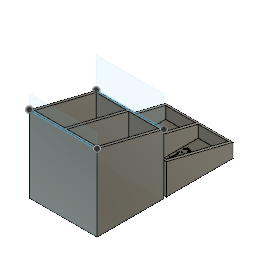
DeckBox (Autodesk Fusion 360 design; units mm, degrees)
Autodesk Fusion 360 part; units mm, degrees
(part 1 of 5)
sketch "Sketch1" plane through (0, 0, 0) normal (0, 0, 1) x (1, 0, 0)
  line L0 (0, 0) -> (35, 0)
  line L1 (35, 0) -> (35, 72)
  line L2 (35, 72) -> (0, 72)
  line L3 (0, 72) -> (0, 0)
  line L4 (38, 0) -> (73, 0)
  line L5 (73, 0) -> (73, 72)
  line L6 (73, 72) -> (38, 72)
  line L7 (38, 72) -> (38, 0)
  line L8 (0, 72) -> (-3, 72)
  line L9 (-3, 72) -> (-3, 75)
  line L10 (-3, 75) -> (0, 75)
  line L11 (0, 75) -> (0, 72)
  line L12 (73, 0) -> (76, 0)
  line L13 (76, 0) -> (76, -3)
  line L14 (76, -3) -> (73, -3)
  line L15 (73, -3) -> (73, 0)
  line L16 (-3, 75) -> (76, 75)
  line L17 (76, 75) -> (76, -3)
  line L18 (76, -3) -> (-3, -3)
  line L19 (-3, -3) -> (-3, 75)
  dimension "d5" = 35
  dimension "d6" = 72
  dimension "d7" = 35
  dimension "d8" = 72
  dimension "d9" = 3
  dimension "d10" = 3
  dimension "d11" = 3
  dimension "d12" = 3
  constraint horizontal L0
  constraint vertical L1
  constraint horizontal L2
  constraint vertical L3
  constraint coincident L0.start L3.end
  constraint horizontal L4
  constraint vertical L5
  constraint horizontal L6
  constraint vertical L7
  constraint horizontal L8
  constraint vertical L9
  constraint horizontal L10
  constraint vertical L11
  constraint horizontal L12
  constraint vertical L13
  constraint horizontal L14
  constraint vertical L15
  constraint horizontal L16
  constraint vertical L17
  constraint horizontal L18
  constraint vertical L19
  measures "d5" distance of L0.start L0.end
  measures "d6" distance of L0.start L2.end
  measures "d7" distance of L4.start L4.end
  measures "d8" distance of L4.start L6.end
  measures "d9" distance of L2.end L8.end
  measures "d10" distance of L2.end L10.end
  measures "d11" distance of L4.end L12.end
  measures "d12" distance of L4.end L14.end
extrude "Extrude1" add sketch "Sketch1" along normal blind 106 makes body 1
sketch "Sketch2" plane through (0, -3, 0) normal (0, -1, 0) x (1, 0, 0)
  line L0 (-3, 0) -> (76, 0)
  line L1 (76, 0) -> (76, 106)
  line L2 (76, 106) -> (-3, 106)
  line L3 (-3, 106) -> (-3, 0)
  line L4 (-3, 106) -> (76, 106)
  line L5 (76, 106) -> (76, 103)
  line L6 (76, 103) -> (-3, 103)
  line L7 (-3, 103) -> (-3, 106)
  line L8 (-3, 0) -> (76, 0)
  line L9 (76, 0) -> (76, 3)
  line L10 (76, 3) -> (-3, 3)
  line L11 (-3, 3) -> (-3, 0)
  dimension "d15" = 3
  dimension "d16" = 3
  constraint horizontal L4
  constraint vertical L5
  constraint horizontal L6
  constraint vertical L7
  constraint coincident L2.end L3.start
  constraint horizontal L8
  constraint vertical L9
  constraint horizontal L10
  constraint vertical L11
  constraint coincident L0.start L3.end
  measures "d15" distance of L2.end L6.end
  measures "d16" distance of L0.start L10.end
extrude "Extrude2" add sketch "Sketch2" against normal blind 78 contours L1 L2 L3 L4 L5 L6 L7 bodies 1
sketch "Sketch3" plane through (0, -3, 0) normal (0, -1, 0) x (1, 0, 0)
  line L0 (-3, 106) -> (-3, 0)
  line L1 (-3, 0) -> (76, 0)
  line L2 (76, 0) -> (76, 106)
  line L3 (76, 106) -> (-3, 106)
  line L4 (-3, 89.5775) -> (76, 89.5775)
  constraint coincident L0 L4.start
  constraint coincident L2 L4.end
  constraint perpendicular L2 L4
sketch "Sketch4" plane through (0, 75, 0) normal (0, 1, 0) x (-1, 0, 0)
  line L0 (-76, 106) -> (-76, 0)
  line L1 (-76, 0) -> (3, 0)
  line L2 (3, 0) -> (3, 106)
  line L3 (3, 106) -> (-76, 106)
  line L4 (-76, 70.2322) -> (3, 70.2322)
  constraint coincident L0 L4.start
  constraint coincident L2 L4.end
  constraint perpendicular L2 L4
ref_plane "WorkPlane1" through (-3, -3, 89.5775) normal (0, -0.240723, -0.970594) x (1, 0, 0)
split "Split1" by plane through (-3, -3, 89.5775) normal (0, -0.240723, -0.970594) bodies 1 makes body 2 at (49.6667, -3, 59.7183)
move_body "Move1" bodies 1 to x (1, 0, 0) y (0, -1, 0) z (0, 0, -1) at (0, 153.0762, 106.2506)
sketch "Sketch5" plane through (76, 0, 0) normal (1, 0, 0) x (0, 1, 0)
  line L0 (75, 70.2322) -> (-3, 89.5775)
  line L1 (-3, 89.5775) -> (-3, 0)
  line L2 (-3, 0) -> (75, 0)
  line L3 (75, 0) -> (75, 70.2322)
  line L4 (-3, 0) -> (75, 0)
  line L5 (75, 0) -> (75, 3)
  line L6 (75, 3) -> (-3, 3)
  line L7 (-3, 3) -> (-3, 0)
  dimension "d19" = 3
  constraint horizontal L4
  constraint vertical L5
  constraint horizontal L6
  constraint vertical L7
  constraint coincident L3 L5.end
  constraint coincident L1.end L2.start
  measures "d19" distance of L1.end L6.end
extrude "Extrude3" add sketch "Sketch5" against normal blind 79 contours L1 L2 L3 L4 L5 L6 L7 bodies 2
sketch "Sketch6" plane through (0, 0, 3.2506) normal (0, 0, 1) x (-1, 0, 0)
  line L0 (-73, -153.0762) -> (-38, -153.0762)
  line L1 (-38, -153.0762) -> (-38, -81.0762)
  line L2 (-38, -81.0762) -> (-73, -81.0762)
  line L3 (-73, -81.0762) -> (-73, -153.0762)
  spline S0 degree 3 poles (-57.9269, -101.8544) (-58.3701, -102.5297) (-58.3595, -103.2367) (-57.8847, -103.6377) knots 0 0 0 0 1 1 1 1
  line L4 (-57.8847, -103.6377) -> (-57.5892, -103.8804)
  line L5 (-57.5892, -103.8804) -> (-58.3384, -104.0703)
  spline S1 degree 3 poles (-58.3384, -104.0703) (-58.75, -104.1758) (-59.2881, -104.3763) (-59.5308, -104.503) knots 0 0 0 0 1 1 1 1
  line L6 (-59.5308, -104.503) -> (-59.9846, -104.7457)
  line L7 (-59.9846, -104.7457) -> (-60.5333, -104.2286)
  spline S2 degree 3 poles (-60.5333, -104.2286) (-61.1031, -103.701) (-61.3036, -103.6166) (-61.388, -103.8382) knots 0 0 0 0 1 1 1 1
  spline S3 degree 3 poles (-61.388, -103.8382) (-61.4196, -103.9437) (-61.4935, -103.9437) (-61.6834, -103.8276) knots 0 0 0 0 1 1 1 1
  spline S4 degree 3 poles (-61.6834, -103.8276) (-62.1688, -103.5322) (-63.5722, -103.3) (-64.5219, -103.3422) knots 0 0 0 0 1 1 1 1
  spline S5 degree 3 poles (-64.5219, -103.3422) (-65.7565, -103.4055) (-65.957, -103.4478) (-66.4318, -103.7538) knots 0 0 0 0 1 1 1 1
  spline S6 degree 3 poles (-66.4318, -103.7538) (-67.0228, -104.1442) (-67.2233, -104.619) (-67.2866, -105.7164) knots 0 0 0 0 1 1 1 1
  spline S7 degree 3 poles (-67.2866, -105.7164) (-67.3077, -106.1174) (-67.4026, -106.2968) (-67.8669, -106.8666) knots 0 0 0 0 1 1 1 1
  spline S8 degree 3 poles (-67.8669, -106.8666) (-68.1729, -107.2465) (-68.4262, -107.6158) (-68.4262, -107.6791) knots 0 0 0 0 1 1 1 1
  spline S9 degree 3 poles (-68.4262, -107.6791) (-68.4262, -107.753) (-68.7216, -108.0379) (-69.0804, -108.3122) knots 0 0 0 0 1 1 1 1
  spline S10 degree 3 poles (-69.0804, -108.3122) (-70.5049, -109.378) (-71.4546, -110.6653) (-71.6446, -111.7733) knots 0 0 0 0 1 1 1 1
  spline S11 degree 3 poles (-71.6446, -111.7733) (-71.7079, -112.1532) (-71.6973, -112.1848) (-71.539, -112.0477) knots 0 0 0 0 1 1 1 1
  spline S12 degree 3 poles (-71.539, -112.0477) (-71.4335, -111.9632) (-71.3913, -111.8155) (-71.423, -111.6889) knots 0 0 0 0 1 1 1 1
  spline S13 degree 3 poles (-71.423, -111.6889) (-71.5601, -111.1613) (-70.3572, -109.589) (-69.1121, -108.671) knots 0 0 0 0 1 1 1 1
  spline S14 degree 3 poles (-69.1121, -108.671) (-68.5317, -108.2489) (-67.3815, -107.563) (-67.3393, -107.6264) knots 0 0 0 0 1 1 1 1
  spline S15 degree 3 poles (-67.3393, -107.6264) (-67.3182, -107.6475) (-67.2444, -107.7846) (-67.1705, -107.9324) knots 0 0 0 0 1 1 1 1
  spline S16 degree 3 poles (-67.1705, -107.9324) (-67.1072, -108.0801) (-66.8856, -108.4811) (-66.7062, -108.8293) knots 0 0 0 0 1 1 1 1
  line L8 (-66.7062, -108.8293) -> (-66.3685, -109.4624)
  line L9 (-66.3685, -109.4624) -> (-67.2655, -110.1588)
  spline S17 degree 3 poles (-67.2655, -110.1588) (-67.7614, -110.5387) (-68.5634, -111.2774) (-69.0382, -111.7839) knots 0 0 0 0 1 1 1 1
  spline S18 degree 3 poles (-69.0382, -111.7839) (-69.513, -112.2904) (-69.9035, -112.6386) (-69.9035, -112.5542) knots 0 0 0 0 1 1 1 1
  spline S19 degree 3 poles (-69.9035, -112.5542) (-69.9035, -112.1954) (-69.4392, -110.9502) (-69.1226, -110.486) knots 0 0 0 0 1 1 1 1
  spline S20 degree 3 poles (-69.1226, -110.486) (-68.8272, -110.0428) (-68.7427, -109.99) (-68.1835, -109.8739) knots 0 0 0 0 1 1 1 1
  spline S21 degree 3 poles (-68.1835, -109.8739) (-67.4871, -109.7368) (-67.2127, -109.5574) (-67.8458, -109.6523) knots 0 0 0 0 1 1 1 1
  spline S22 degree 3 poles (-67.8458, -109.6523) (-69.1543, -109.8528) (-70.3467, -110.4015) (-71.0536, -111.1402) knots 0 0 0 0 1 1 1 1
  spline S23 degree 3 poles (-71.0536, -111.1402) (-71.5601, -111.6678) (-71.4124, -111.71) (-70.8531, -111.2035) knots 0 0 0 0 1 1 1 1
  spline S24 degree 3 poles (-70.8531, -111.2035) (-70.4733, -110.8553) (-69.3864, -110.2116) (-69.3126, -110.2855) knots 0 0 0 0 1 1 1 1
  spline S25 degree 3 poles (-69.3126, -110.2855) (-69.2914, -110.296) (-69.4181, -110.5915) (-69.5869, -110.9397) knots 0 0 0 0 1 1 1 1
  spline S26 degree 3 poles (-69.5869, -110.9397) (-69.7557, -111.2879) (-69.9351, -111.8577) (-69.9984, -112.1954) knots 0 0 0 0 1 1 1 1
  spline S27 degree 3 poles (-69.9984, -112.1954) (-70.0934, -112.6913) (-70.2728, -113.0712) (-70.9059, -114.0314) knots 0 0 0 0 1 1 1 1
  spline S28 degree 3 poles (-70.9059, -114.0314) (-71.3385, -114.6962) (-71.6973, -115.3399) (-71.6973, -115.4665) knots 0 0 0 0 1 1 1 1
  spline S29 degree 3 poles (-71.6973, -115.4665) (-71.6973, -115.6353) (-71.634, -115.5826) (-71.4441, -115.2449) knots 0 0 0 0 1 1 1 1
  spline S30 degree 3 poles (-71.4441, -115.2449) (-70.4944, -113.5777) (-68.3734, -111.1402) (-66.9172, -110.0533) knots 0 0 0 0 1 1 1 1
  spline S31 degree 3 poles (-66.9172, -110.0533) (-66.4107, -109.6735) (-66.2841, -109.6207) (-66.1575, -109.7262) knots 0 0 0 0 1 1 1 1
  spline S32 degree 3 poles (-66.1575, -109.7262) (-66.0098, -109.8423) (-66.0098, -109.8845) (-66.1786, -110.0639) knots 0 0 0 0 1 1 1 1
  spline S33 degree 3 poles (-66.1786, -110.0639) (-66.3369, -110.2433) (-66.3474, -110.2855) (-66.2103, -110.3699) knots 0 0 0 0 1 1 1 1
  spline S34 degree 3 poles (-66.2103, -110.3699) (-65.746, -110.6442) (-65.7565, -110.602) (-66.0836, -111.6572) knots 0 0 0 0 1 1 1 1
  spline S35 degree 3 poles (-66.0836, -111.6572) (-66.7379, -113.6938) (-67.7086, -115.878) (-68.194, -116.3951) knots 0 0 0 0 1 1 1 1
  spline S36 degree 3 poles (-68.194, -116.3951) (-68.3418, -116.5639) (-68.4367, -116.6906) (-68.3945, -116.6906) knots 0 0 0 0 1 1 1 1
  spline S37 degree 3 poles (-68.3945, -116.6906) (-68.194, -116.6906) (-67.3499, -116.2157) (-66.9911, -115.9097) knots 0 0 0 0 1 1 1 1
  line L10 (-66.9911, -115.9097) -> (-66.5796, -115.5615)
  line L11 (-66.5796, -115.5615) -> (-66.5901, -117.2076)
  spline S38 degree 3 poles (-66.5901, -117.2076) (-66.6112, -120.0039) (-66.8961, -120.9958) (-67.8458, -121.6289) knots 0 0 0 0 1 1 1 1
  spline S39 degree 3 poles (-67.8458, -121.6289) (-68.2046, -121.861) (-68.2785, -121.956) (-68.1518, -122.0088) knots 0 0 0 0 1 1 1 1
  spline S40 degree 3 poles (-68.1518, -122.0088) (-67.8458, -122.1248) (-67.1072, -122.0615) (-66.5585, -121.8716) knots 0 0 0 0 1 1 1 1
  line L12 (-66.5585, -121.8716) -> (-66.0098, -121.6922)
  line L13 (-66.0098, -121.6922) -> (-66.2841, -122.2198)
  spline S41 degree 3 poles (-66.2841, -122.2198) (-66.4318, -122.5153) (-66.6112, -122.7896) (-66.6745, -122.8318) knots 0 0 0 0 1 1 1 1
  spline S42 degree 3 poles (-66.6745, -122.8318) (-66.9911, -123.0429) (-66.1153, -122.8846) (-65.7354, -122.663) knots 0 0 0 0 1 1 1 1
  line L14 (-65.7354, -122.663) -> (-65.3028, -122.3992)
  line L15 (-65.3028, -122.3992) -> (-65.1762, -123.2117)
  spline S43 degree 3 poles (-65.1762, -123.2117) (-65.1128, -123.6549) (-64.8807, -124.478) (-64.6697, -125.0267) knots 0 0 0 0 1 1 1 1
  spline S44 degree 3 poles (-64.6697, -125.0267) (-64.2054, -126.2612) (-64.0154, -126.926) (-63.931, -127.6119) knots 0 0 0 0 1 1 1 1
  spline S45 degree 3 poles (-63.931, -127.6119) (-63.8783, -128.1078) (-63.8994, -128.1712) (-64.3214, -128.7515) knots 0 0 0 0 1 1 1 1
  spline S46 degree 3 poles (-64.3214, -128.7515) (-64.5641, -129.0786) (-64.8068, -129.353) (-64.849, -129.353) knots 0 0 0 0 1 1 1 1
  spline S47 degree 3 poles (-64.849, -129.353) (-65.0284, -129.353) (-65.039, -129.1631) (-64.8913, -128.6671) knots 0 0 0 0 1 1 1 1
  spline S48 degree 3 poles (-64.8913, -128.6671) (-64.7119, -128.0762) (-64.6697, -127.116) (-64.849, -127.5486) knots 0 0 0 0 1 1 1 1
  spline S49 degree 3 poles (-64.849, -127.5486) (-64.9018, -127.6858) (-65.2817, -128.129) (-65.6827, -128.5299) knots 0 0 0 0 1 1 1 1
  spline S50 degree 3 poles (-65.6827, -128.5299) (-66.2525, -129.0997) (-66.4635, -129.2475) (-66.6218, -129.1947) knots 0 0 0 0 1 1 1 1
  spline S51 degree 3 poles (-66.6218, -129.1947) (-66.9067, -129.1103) (-67.6664, -129.3108) (-68.0358, -129.5746) knots 0 0 0 0 1 1 1 1
  spline S52 degree 3 poles (-68.0358, -129.5746) (-68.2046, -129.7012) (-68.3629, -129.7751) (-68.384, -129.7434) knots 0 0 0 0 1 1 1 1
  spline S53 degree 3 poles (-68.384, -129.7434) (-68.4473, -129.6907) (-68.1202, -128.9415) (-67.4026, -127.4747) knots 0 0 0 0 1 1 1 1
  spline S54 degree 3 poles (-67.4026, -127.4747) (-67.0755, -126.8205) (-66.8434, -126.2612) (-66.875, -126.2296) knots 0 0 0 0 1 1 1 1
  spline S55 degree 3 poles (-66.875, -126.2296) (-66.9067, -126.1979) (-67.1283, -126.5884) (-67.3815, -127.0949) knots 0 0 0 0 1 1 1 1
  spline S56 degree 3 poles (-67.3815, -127.0949) (-67.9513, -128.2872) (-68.4684, -128.7937) (-69.5025, -129.2264) knots 0 0 0 0 1 1 1 1
  spline S57 degree 3 poles (-69.5025, -129.2264) (-70.5577, -129.6695) (-70.6632, -129.6484) (-70.0406, -129.1525) knots 0 0 0 0 1 1 1 1
  spline S58 degree 3 poles (-70.0406, -129.1525) (-69.7663, -128.9309) (-69.4075, -128.6143) (-69.2598, -128.4455) knots 0 0 0 0 1 1 1 1
  spline S59 degree 3 poles (-69.2598, -128.4455) (-68.8377, -127.9707) (-68.1624, -126.8311) (-67.9091, -126.1452) knots 0 0 0 0 1 1 1 1
  spline S60 degree 3 poles (-67.9091, -126.1452) (-67.7825, -125.797) (-67.6453, -125.4698) (-67.6031, -125.4065) knots 0 0 0 0 1 1 1 1
  spline S61 degree 3 poles (-67.6031, -125.4065) (-67.5715, -125.3432) (-67.5293, -125.2377) (-67.5187, -125.1849) knots 0 0 0 0 1 1 1 1
  spline S62 degree 3 poles (-67.5187, -125.1849) (-67.5082, -125.1216) (-67.3815, -124.7101) (-67.2233, -124.2564) knots 0 0 0 0 1 1 1 1
  spline S63 degree 3 poles (-67.2233, -124.2564) (-67.0755, -123.8026) (-66.9067, -123.2328) (-66.8434, -122.9796) knots 0 0 0 0 1 1 1 1
  spline S64 degree 3 poles (-66.8434, -122.9796) (-66.7906, -122.7369) (-66.7168, -122.452) (-66.6745, -122.357) knots 0 0 0 0 1 1 1 1
  spline S65 degree 3 poles (-66.6745, -122.357) (-66.6429, -122.262) (-66.6534, -122.1776) (-66.7062, -122.1776) knots 0 0 0 0 1 1 1 1
  spline S66 degree 3 poles (-66.7062, -122.1776) (-66.759, -122.1776) (-66.8856, -122.5469) (-66.9911, -122.9901) knots 0 0 0 0 1 1 1 1
  spline S67 degree 3 poles (-66.9911, -122.9901) (-67.0966, -123.4439) (-67.2233, -123.8554) (-67.2655, -123.9187) knots 0 0 0 0 1 1 1 1
  spline S68 degree 3 poles (-67.2655, -123.9187) (-67.2971, -123.9715) (-67.4871, -124.4991) (-67.6875, -125.0794) knots 0 0 0 0 1 1 1 1
  spline S69 degree 3 poles (-67.6875, -125.0794) (-68.0674, -126.2401) (-68.4895, -127.1687) (-68.8799, -127.6858) knots 0 0 0 0 1 1 1 1
  spline S70 degree 3 poles (-68.8799, -127.6858) (-69.0171, -127.8757) (-69.1648, -128.1184) (-69.1965, -128.2134) knots 0 0 0 0 1 1 1 1
  spline S71 degree 3 poles (-69.1965, -128.2134) (-69.2809, -128.4455) (-70.6738, -129.4691) (-71.2436, -129.7223) knots 0 0 0 0 1 1 1 1
  spline S72 degree 3 poles (-71.2436, -129.7223) (-71.4968, -129.8278) (-71.6973, -129.9545) (-71.6973, -130.0072) knots 0 0 0 0 1 1 1 1
  spline S73 degree 3 poles (-71.6973, -130.0072) (-71.6973, -130.1338) (-71.5179, -130.1127) (-71.1908, -129.9439) knots 0 0 0 0 1 1 1 1
  spline S74 degree 3 poles (-71.1908, -129.9439) (-71.0325, -129.87) (-70.6738, -129.7645) (-70.3889, -129.7223) knots 0 0 0 0 1 1 1 1
  spline S75 degree 3 poles (-70.3889, -129.7223) (-69.7346, -129.6273) (-68.901, -129.2686) (-68.4367, -128.8676) knots 0 0 0 0 1 1 1 1
  line L16 (-68.4367, -128.8676) -> (-68.0674, -128.5616)
  line L17 (-68.0674, -128.5616) -> (-68.3734, -129.1314)
  line L18 (-68.3734, -129.1314) -> (-68.6794, -129.6907)
  line L19 (-68.6794, -129.6907) -> (-69.1332, -129.6273)
  spline S76 degree 3 poles (-69.1332, -129.6273) (-69.608, -129.564) (-69.6713, -129.6273) (-69.4919, -129.9756) knots 0 0 0 0 1 1 1 1
  spline S77 degree 3 poles (-69.4919, -129.9756) (-69.4075, -130.1338) (-69.4708, -130.2077) (-69.8929, -130.4398) knots 0 0 0 0 1 1 1 1
  spline S78 degree 3 poles (-69.8929, -130.4398) (-70.2939, -130.6509) (-71.6973, -131.9171) (-71.6973, -132.0649) knots 0 0 0 0 1 1 1 1
  spline S79 degree 3 poles (-71.6973, -132.0649) (-71.6973, -132.2231) (-71.3913, -131.991) (-70.832, -131.4106) knots 0 0 0 0 1 1 1 1
  spline S80 degree 3 poles (-70.832, -131.4106) (-70.3467, -130.9041) (-70.0195, -130.672) (-69.6186, -130.5243) knots 0 0 0 0 1 1 1 1
  spline S81 degree 3 poles (-69.6186, -130.5243) (-69.1543, -130.3554) (-69.0488, -130.3449) (-68.9432, -130.4715) knots 0 0 0 0 1 1 1 1
  spline S82 degree 3 poles (-68.9432, -130.4715) (-68.8799, -130.5559) (-68.7216, -130.6192) (-68.595, -130.6192) knots 0 0 0 0 1 1 1 1
  spline S83 degree 3 poles (-68.595, -130.6192) (-68.4051, -130.6192) (-68.4156, -130.5981) (-68.69, -130.4187) knots 0 0 0 0 1 1 1 1
  spline S84 degree 3 poles (-68.69, -130.4187) (-68.8588, -130.3132) (-69.1015, -130.1233) (-69.207, -129.9967) knots 0 0 0 0 1 1 1 1
  line L20 (-69.207, -129.9967) -> (-69.4075, -129.7751)
  line L21 (-69.4075, -129.7751) -> (-68.8905, -129.8384)
  spline S85 degree 3 poles (-68.8905, -129.8384) (-68.6056, -129.8806) (-68.3523, -129.9228) (-68.3312, -129.9545) knots 0 0 0 0 1 1 1 1
  spline S86 degree 3 poles (-68.3312, -129.9545) (-68.2996, -129.9756) (-68.1835, -129.9017) (-68.0674, -129.7856) knots 0 0 0 0 1 1 1 1
  spline S87 degree 3 poles (-68.0674, -129.7856) (-67.5609, -129.3319) (-66.5585, -129.258) (-65.862, -129.6168) knots 0 0 0 0 1 1 1 1
  line L22 (-65.862, -129.6168) -> (-65.5771, -129.7645)
  line L23 (-65.5771, -129.7645) -> (-65.6404, -129.3424)
  line L24 (-65.6404, -129.3424) -> (-65.7143, -128.9204)
  line L25 (-65.7143, -128.9204) -> (-65.3344, -129.1631)
  spline S88 degree 3 poles (-65.3344, -129.1631) (-65.1234, -129.3002) (-64.9546, -129.4269) (-64.9546, -129.4585) knots 0 0 0 0 1 1 1 1
  spline S89 degree 3 poles (-64.9546, -129.4585) (-64.944, -129.5746) (-65.8726, -130.176) (-66.2419, -130.3027) knots 0 0 0 0 1 1 1 1
  spline S90 degree 3 poles (-66.2419, -130.3027) (-66.7906, -130.4715) (-66.6323, -130.6614) (-65.9887, -130.5876) knots 0 0 0 0 1 1 1 1
  spline S91 degree 3 poles (-65.9887, -130.5876) (-65.4822, -130.5243) (-64.733, -130.2077) (-64.3848, -129.9017) knots 0 0 0 0 1 1 1 1
  spline S92 degree 3 poles (-64.3848, -129.9017) (-64.2687, -129.7962) (-64.3425, -130.0494) (-64.6063, -130.6298) knots 0 0 0 0 1 1 1 1
  spline S93 degree 3 poles (-64.6063, -130.6298) (-64.8385, -131.1152) (-65.0495, -131.59) (-65.0812, -131.685) knots 0 0 0 0 1 1 1 1
  spline S94 degree 3 poles (-65.0812, -131.685) (-65.1128, -131.78) (-65.3344, -131.9488) (-65.5666, -132.0543) knots 0 0 0 0 1 1 1 1
  spline S95 degree 3 poles (-65.5666, -132.0543) (-65.7987, -132.1704) (-65.9992, -132.2865) (-65.9992, -132.3287) knots 0 0 0 0 1 1 1 1
  spline S96 degree 3 poles (-65.9992, -132.3287) (-65.9992, -132.4025) (-65.862, -132.3603) (-65.2078, -132.086) knots 0 0 0 0 1 1 1 1
  spline S97 degree 3 poles (-65.2078, -132.086) (-65.0284, -132.0121) (-64.8385, -131.9699) (-64.7857, -131.9804) knots 0 0 0 0 1 1 1 1
  spline S98 degree 3 poles (-64.7857, -131.9804) (-64.7224, -132.0015) (-64.7119, -131.9699) (-64.7541, -131.9277) knots 0 0 0 0 1 1 1 1
  spline S99 degree 3 poles (-64.7541, -131.9277) (-64.7963, -131.8855) (-64.5958, -131.6006) (-64.3109, -131.2946) knots 0 0 0 0 1 1 1 1
  spline S100 degree 3 poles (-64.3109, -131.2946) (-63.9521, -130.8936) (-63.7516, -130.5559) (-63.6356, -130.1444) knots 0 0 0 0 1 1 1 1
  spline S101 degree 3 poles (-63.6356, -130.1444) (-63.5406, -129.8278) (-63.4351, -129.4902) (-63.3929, -129.3952) knots 0 0 0 0 1 1 1 1
  spline S102 degree 3 poles (-63.3929, -129.3952) (-63.3507, -129.2791) (-63.3718, -129.2369) (-63.4351, -129.2791) knots 0 0 0 0 1 1 1 1
  spline S103 degree 3 poles (-63.4351, -129.2791) (-63.4984, -129.3213) (-63.625, -129.6379) (-63.7305, -130.0072) knots 0 0 0 0 1 1 1 1
  spline S104 degree 3 poles (-63.7305, -130.0072) (-63.8677, -130.5137) (-64.026, -130.7775) (-64.427, -131.189) knots 0 0 0 0 1 1 1 1
  line L26 (-64.427, -131.189) -> (-64.944, -131.7272)
  line L27 (-64.944, -131.7272) -> (-64.6275, -131.073)
  spline S105 degree 3 poles (-64.6275, -131.073) (-64.4586, -130.7142) (-64.2476, -130.2394) (-64.1526, -130.0178) knots 0 0 0 0 1 1 1 1
  spline S106 degree 3 poles (-64.1526, -130.0178) (-63.9521, -129.5324) (-63.4773, -129.0153) (-63.319, -129.1103) knots 0 0 0 0 1 1 1 1
  spline S107 degree 3 poles (-63.319, -129.1103) (-63.2557, -129.1419) (-63.2346, -129.1419) (-63.2768, -129.0892) knots 0 0 0 0 1 1 1 1
  spline S108 degree 3 poles (-63.2768, -129.0892) (-63.319, -129.047) (-63.2557, -128.8254) (-63.1396, -128.6038) knots 0 0 0 0 1 1 1 1
  spline S109 degree 3 poles (-63.1396, -128.6038) (-63.0235, -128.3716) (-62.9813, -128.1923) (-63.0446, -128.1923) knots 0 0 0 0 1 1 1 1
  spline S110 degree 3 poles (-63.0446, -128.1923) (-63.0974, -128.1923) (-63.1502, -128.2661) (-63.1502, -128.3611) knots 0 0 0 0 1 1 1 1
  spline S111 degree 3 poles (-63.1502, -128.3611) (-63.1502, -128.4561) (-63.4456, -128.8254) (-63.8149, -129.1842) knots 0 0 0 0 1 1 1 1
  spline S112 degree 3 poles (-63.8149, -129.1842) (-64.4903, -129.8595) (-65.345, -130.366) (-65.9992, -130.461) knots 0 0 0 0 1 1 1 1
  line L28 (-65.9992, -130.461) -> (-66.3685, -130.5137)
  line L29 (-66.3685, -130.5137) -> (-66.052, -130.3976)
  spline S113 degree 3 poles (-66.052, -130.3976) (-64.9546, -129.9756) (-63.8888, -128.7199) (-63.3084, -127.1898) knots 0 0 0 0 1 1 1 1
  spline S114 degree 3 poles (-63.3084, -127.1898) (-62.8336, -125.9025) (-62.5382, -123.5705) (-62.8442, -123.3911) knots 0 0 0 0 1 1 1 1
  spline S115 degree 3 poles (-62.8442, -123.3911) (-62.918, -123.3383) (-62.9286, -123.4333) (-62.8864, -123.676) knots 0 0 0 0 1 1 1 1
  spline S116 degree 3 poles (-62.8864, -123.676) (-62.7808, -124.2353) (-63.0235, -125.8181) (-63.3929, -126.9155) knots 0 0 0 0 1 1 1 1
  line L30 (-63.3929, -126.9155) -> (-63.72, -127.9285)
  line L31 (-63.72, -127.9285) -> (-63.7938, -127.4009)
  spline S117 degree 3 poles (-63.7938, -127.4009) (-63.8255, -127.1054) (-63.9943, -126.5145) (-64.1526, -126.0819) knots 0 0 0 0 1 1 1 1
  spline S118 degree 3 poles (-64.1526, -126.0819) (-64.5852, -124.8789) (-64.9229, -123.7288) (-65.0601, -122.9796) knots 0 0 0 0 1 1 1 1
  spline S119 degree 3 poles (-65.0601, -122.9796) (-65.1656, -122.3253) (-65.1656, -122.2937) (-64.8807, -121.8716) knots 0 0 0 0 1 1 1 1
  spline S120 degree 3 poles (-64.8807, -121.8716) (-64.7224, -121.6289) (-64.6275, -121.4073) (-64.6591, -121.3651) knots 0 0 0 0 1 1 1 1
  spline S121 degree 3 poles (-64.6591, -121.3651) (-64.7013, -121.3334) (-64.7646, -121.3968) (-64.8068, -121.5023) knots 0 0 0 0 1 1 1 1
  spline S122 degree 3 poles (-64.8068, -121.5023) (-64.9335, -121.8294) (-65.3872, -122.2831) (-65.8726, -122.568) knots 0 0 0 0 1 1 1 1
  spline S123 degree 3 poles (-65.8726, -122.568) (-66.1258, -122.7158) (-66.3369, -122.8213) (-66.358, -122.8002) knots 0 0 0 0 1 1 1 1
  spline S124 degree 3 poles (-66.358, -122.8002) (-66.3791, -122.7791) (-66.2208, -122.3886) (-65.9992, -121.9349) knots 0 0 0 0 1 1 1 1
  spline S125 degree 3 poles (-65.9992, -121.9349) (-65.7882, -121.4917) (-65.6193, -121.1224) (-65.6404, -121.1224) knots 0 0 0 0 1 1 1 1
  spline S126 degree 3 poles (-65.6404, -121.1224) (-65.6616, -121.1224) (-65.7987, -121.2385) (-65.957, -121.3862) knots 0 0 0 0 1 1 1 1
  spline S127 degree 3 poles (-65.957, -121.3862) (-66.2525, -121.6606) (-66.7062, -121.8188) (-67.4343, -121.8927) knots 0 0 0 0 1 1 1 1
  line L32 (-67.4343, -121.8927) -> (-67.8669, -121.9455)
  line L33 (-67.8669, -121.9455) -> (-67.4343, -121.5023)
  spline S128 degree 3 poles (-67.4343, -121.5023) (-66.8961, -120.9747) (-66.5163, -120.2993) (-66.2314, -119.413) knots 0 0 0 0 1 1 1 1
  spline S129 degree 3 poles (-66.2314, -119.413) (-65.8937, -118.3683) (-65.7882, -117.7985) (-65.7987, -117.197) knots 0 0 0 0 1 1 1 1
  spline S130 degree 3 poles (-65.7987, -117.197) (-65.8093, -116.6906) (-65.8198, -116.7222) (-65.957, -117.5875) knots 0 0 0 0 1 1 1 1
  spline S131 degree 3 poles (-65.957, -117.5875) (-66.0309, -118.1045) (-66.2103, -118.8643) (-66.358, -119.2758) knots 0 0 0 0 1 1 1 1
  spline S132 degree 3 poles (-66.358, -119.2758) (-66.5057, -119.6768) (-66.6007, -119.8456) (-66.5585, -119.6451) knots 0 0 0 0 1 1 1 1
  spline S133 degree 3 poles (-66.5585, -119.6451) (-66.4318, -118.9381) (-66.4213, -118.7376) (-66.4318, -117.6402) knots 0 0 0 0 1 1 1 1
  spline S134 degree 3 poles (-66.4318, -117.6402) (-66.4635, -115.7092) (-66.4318, -115.3927) (-66.2314, -115.1077) knots 0 0 0 0 1 1 1 1
  spline S135 degree 3 poles (-66.2314, -115.1077) (-65.9359, -114.7173) (-65.7671, -114.3691) (-65.862, -114.3691) knots 0 0 0 0 1 1 1 1
  spline S136 degree 3 poles (-65.862, -114.3691) (-65.9148, -114.3691) (-66.0414, -114.5274) (-66.1469, -114.7068) knots 0 0 0 0 1 1 1 1
  spline S137 degree 3 poles (-66.1469, -114.7068) (-66.453, -115.2449) (-67.8986, -116.5428) (-67.8986, -116.279) knots 0 0 0 0 1 1 1 1
  spline S138 degree 3 poles (-67.8986, -116.279) (-67.8986, -116.2263) (-67.8458, -116.1418) (-67.7931, -116.1102) knots 0 0 0 0 1 1 1 1
  spline S139 degree 3 poles (-67.7931, -116.1102) (-67.6137, -116.0047) (-66.8117, -114.2108) (-66.3158, -112.8391) knots 0 0 0 0 1 1 1 1
  spline S140 degree 3 poles (-66.3158, -112.8391) (-65.4294, -110.3382) (-64.9335, -109.1353) (-64.638, -108.7027) knots 0 0 0 0 1 1 1 1
  spline S141 degree 3 poles (-64.638, -108.7027) (-64.1104, -107.9218) (-63.2662, -106.9299) (-62.802, -106.5501) knots 0 0 0 0 1 1 1 1
  spline S142 degree 3 poles (-62.802, -106.5501) (-62.2005, -106.0436) (-61.1558, -105.3577) (-61.0925, -105.421) knots 0 0 0 0 1 1 1 1
  spline S143 degree 3 poles (-61.0925, -105.421) (-61.0609, -105.4526) (-61.2403, -105.6109) (-61.4829, -105.7692) knots 0 0 0 0 1 1 1 1
  spline S144 degree 3 poles (-61.4829, -105.7692) (-62.3166, -106.3179) (-64.0471, -108.2489) (-63.7094, -108.2489) knots 0 0 0 0 1 1 1 1
  spline S145 degree 3 poles (-63.7094, -108.2489) (-63.6567, -108.2489) (-63.53, -108.0906) (-63.414, -107.9007) knots 0 0 0 0 1 1 1 1
  spline S146 degree 3 poles (-63.414, -107.9007) (-63.1713, -107.4892) (-62.3799, -106.6978) (-61.4935, -105.9802) knots 0 0 0 0 1 1 1 1
  spline S147 degree 3 poles (-61.4935, -105.9802) (-61.0398, -105.6215) (-60.8815, -105.4315) (-60.9659, -105.3682) knots 0 0 0 0 1 1 1 1
  spline S148 degree 3 poles (-60.9659, -105.3682) (-61.0503, -105.3049) (-61.0292, -105.2944) (-60.9131, -105.3366) knots 0 0 0 0 1 1 1 1
  spline S149 degree 3 poles (-60.9131, -105.3366) (-60.8076, -105.3682) (-60.4277, -105.2099) (-60.0162, -104.9672) knots 0 0 0 0 1 1 1 1
  spline S150 degree 3 poles (-60.0162, -104.9672) (-59.6258, -104.7351) (-58.961, -104.4502) (-58.56, -104.3341) knots 0 0 0 0 1 1 1 1
  spline S151 degree 3 poles (-58.56, -104.3341) (-57.3571, -103.9754) (-57.3571, -103.9754) (-57.7264, -104.313) knots 0 0 0 0 1 1 1 1
  spline S152 degree 3 poles (-57.7264, -104.313) (-58.1274, -104.6718) (-58.6761, -105.3999) (-58.5495, -105.3999) knots 0 0 0 0 1 1 1 1
  spline S153 degree 3 poles (-58.5495, -105.3999) (-58.4967, -105.3999) (-58.3173, -105.231) (-58.1591, -105.0306) knots 0 0 0 0 1 1 1 1
  spline S154 degree 3 poles (-58.1591, -105.0306) (-57.6737, -104.4291) (-56.8717, -103.8487) (-56.4074, -103.7643) knots 0 0 0 0 1 1 1 1
  spline S155 degree 3 poles (-56.4074, -103.7643) (-56.0592, -103.7116) (-55.8587, -103.7538) (-55.3733, -103.9859) knots 0 0 0 0 1 1 1 1
  spline S156 degree 3 poles (-55.3733, -103.9859) (-54.5292, -104.3869) (-54.5081, -104.3974) (-54.8457, -104.0914) knots 0 0 0 0 1 1 1 1
  spline S157 degree 3 poles (-54.8457, -104.0914) (-55.1412, -103.8171) (-55.1412, -103.8171) (-54.8985, -103.8171) knots 0 0 0 0 1 1 1 1
  spline S158 degree 3 poles (-54.8985, -103.8171) (-54.5292, -103.8171) (-53.2524, -104.102) (-52.5981, -104.3236) knots 0 0 0 0 1 1 1 1
  spline S159 degree 3 poles (-52.5981, -104.3236) (-51.3108, -104.7668) (-50.1712, -105.5054) (-48.9788, -106.6556) knots 0 0 0 0 1 1 1 1
  spline S160 degree 3 poles (-48.9788, -106.6556) (-47.8814, -107.7108) (-47.1322, -108.7976) (-46.3619, -110.4226) knots 0 0 0 0 1 1 1 1
  spline S161 degree 3 poles (-46.3619, -110.4226) (-45.6866, -111.8472) (-45.3489, -112.4064) (-44.5997, -113.2928) knots 0 0 0 0 1 1 1 1
  spline S162 degree 3 poles (-44.5997, -113.2928) (-44.1671, -113.8098) (-44.1565, -113.8415) (-44.4414, -113.7149) knots 0 0 0 0 1 1 1 1
  spline S163 degree 3 poles (-44.4414, -113.7149) (-44.5997, -113.6516) (-45.0851, -113.3667) (-45.4966, -113.0923) knots 0 0 0 0 1 1 1 1
  spline S164 degree 3 poles (-45.4966, -113.0923) (-46.2775, -112.5858) (-46.4674, -112.5436) (-46.0137, -112.9762) knots 0 0 0 0 1 1 1 1
  spline S165 degree 3 poles (-46.0137, -112.9762) (-45.7393, -113.2295) (-45.5283, -113.9787) (-45.5283, -114.7068) knots 0 0 0 0 1 1 1 1
  spline S166 degree 3 poles (-45.5283, -114.7068) (-45.5283, -115.3399) (-45.2328, -116.8488) (-45.0007, -117.387) knots 0 0 0 0 1 1 1 1
  spline S167 degree 3 poles (-45.0007, -117.387) (-44.6525, -118.1995) (-44.8952, -117.8935) (-45.3172, -116.9755) knots 0 0 0 0 1 1 1 1
  spline S168 degree 3 poles (-45.3172, -116.9755) (-45.5388, -116.5006) (-45.8237, -115.762) (-45.9398, -115.3293) knots 0 0 0 0 1 1 1 1
  spline S169 degree 3 poles (-45.9398, -115.3293) (-46.172, -114.5063) (-46.3408, -114.1686) (-46.2142, -114.7912) knots 0 0 0 0 1 1 1 1
  spline S170 degree 3 poles (-46.2142, -114.7912) (-46.077, -115.5193) (-45.7077, -116.5428) (-45.2961, -117.3342) knots 0 0 0 0 1 1 1 1
  spline S171 degree 3 poles (-45.2961, -117.3342) (-44.8846, -118.1467) (-44.0088, -119.1597) (-43.6184, -119.2758) knots 0 0 0 0 1 1 1 1
  spline S172 degree 3 poles (-43.6184, -119.2758) (-43.2174, -119.4024) (-43.3018, -119.2441) (-43.7872, -118.9698) knots 0 0 0 0 1 1 1 1
  spline S173 degree 3 poles (-43.7872, -118.9698) (-44.0827, -118.7904) (-44.3359, -118.5372) (-44.4731, -118.2734) knots 0 0 0 0 1 1 1 1
  spline S174 degree 3 poles (-44.4731, -118.2734) (-44.8318, -117.5769) (-45.2117, -116.0574) (-45.3594, -114.7701) knots 0 0 0 0 1 1 1 1
  spline S175 degree 3 poles (-45.3594, -114.7701) (-45.4439, -114.0948) (-45.5388, -113.4827) (-45.581, -113.4194) knots 0 0 0 0 1 1 1 1
  spline S176 degree 3 poles (-45.581, -113.4194) (-45.6232, -113.3561) (-45.4122, -113.4194) (-45.1273, -113.5672) knots 0 0 0 0 1 1 1 1
  spline S177 degree 3 poles (-45.1273, -113.5672) (-44.6208, -113.8204) (-43.65, -114.1053) (-43.5551, -114.0209) knots 0 0 0 0 1 1 1 1
  spline S178 degree 3 poles (-43.5551, -114.0209) (-43.5339, -113.9998) (-43.7028, -113.8521) (-43.9244, -113.6938) knots 0 0 0 0 1 1 1 1
  spline S179 degree 3 poles (-43.9244, -113.6938) (-44.4309, -113.3456) (-45.3067, -112.2059) (-45.7499, -111.3196) knots 0 0 0 0 1 1 1 1
  line L34 (-45.7499, -111.3196) -> (-46.077, -110.6337)
  line L35 (-46.077, -110.6337) -> (-45.8554, -110.4543)
  spline S180 degree 3 poles (-45.8554, -110.4543) (-45.5916, -110.2327) (-45.5705, -110.085) (-45.8132, -110.0006) knots 0 0 0 0 1 1 1 1
  spline S181 degree 3 poles (-45.8132, -110.0006) (-45.9715, -109.9373) (-45.9715, -109.9161) (-45.8132, -109.7579) knots 0 0 0 0 1 1 1 1
  spline S182 degree 3 poles (-45.8132, -109.7579) (-45.6549, -109.5996) (-45.6021, -109.6207) (-45.0323, -110.0428) knots 0 0 0 0 1 1 1 1
  spline S183 degree 3 poles (-45.0323, -110.0428) (-44.2409, -110.6337) (-42.3838, -112.4486) (-41.719, -113.2717) knots 0 0 0 0 1 1 1 1
  spline S184 degree 3 poles (-41.719, -113.2717) (-41.4341, -113.6305) (-40.9381, -114.3375) (-40.6216, -114.8439) knots 0 0 0 0 1 1 1 1
  spline S185 degree 3 poles (-40.6216, -114.8439) (-40.2839, -115.3821) (-40.0412, -115.6881) (-40.0412, -115.5615) knots 0 0 0 0 1 1 1 1
  spline S186 degree 3 poles (-40.0412, -115.5615) (-40.0412, -115.456) (-40.3894, -114.8334) (-40.8221, -114.1792) knots 0 0 0 0 1 1 1 1
  spline S187 degree 3 poles (-40.8221, -114.1792) (-41.3286, -113.4089) (-41.624, -112.8707) (-41.6557, -112.6069) knots 0 0 0 0 1 1 1 1
  spline S188 degree 3 poles (-41.6557, -112.6069) (-41.7401, -112.0055) (-41.8984, -111.4673) (-42.1411, -110.9714) knots 0 0 0 0 1 1 1 1
  spline S189 degree 3 poles (-42.1411, -110.9714) (-42.2572, -110.7287) (-42.3416, -110.5071) (-42.3205, -110.486) knots 0 0 0 0 1 1 1 1
  spline S190 degree 3 poles (-42.3205, -110.486) (-42.2994, -110.4649) (-42.0145, -110.5704) (-41.6979, -110.7287) knots 0 0 0 0 1 1 1 1
  spline S191 degree 3 poles (-41.6979, -110.7287) (-41.3286, -110.8975) (-40.9065, -111.2246) (-40.5583, -111.6045) knots 0 0 0 0 1 1 1 1
  line L36 (-40.5583, -111.6045) -> (-40.0096, -112.1954)
  line L37 (-40.0096, -112.1954) -> (-40.094, -111.8366)
  spline S192 degree 3 poles (-40.094, -111.8366) (-40.2734, -110.9714) (-41.2231, -109.7579) (-42.7848, -108.4072) knots 0 0 0 0 1 1 1 1
  spline S193 degree 3 poles (-42.7848, -108.4072) (-43.1857, -108.0484) (-44.2515, -106.6872) (-44.4203, -106.3179) knots 0 0 0 0 1 1 1 1
  spline S194 degree 3 poles (-44.4203, -106.3179) (-44.4731, -106.1913) (-44.5469, -106.0647) (-44.5891, -106.033) knots 0 0 0 0 1 1 1 1
  spline S195 degree 3 poles (-44.5891, -106.033) (-44.6208, -106.0013) (-44.6947, -105.6953) (-44.7263, -105.3471) knots 0 0 0 0 1 1 1 1
  spline S196 degree 3 poles (-44.7263, -105.3471) (-44.8213, -104.5979) (-45.0851, -103.9648) (-45.4333, -103.6377) knots 0 0 0 0 1 1 1 1
  spline S197 degree 3 poles (-45.4333, -103.6377) (-46.1931, -102.9413) (-48.6833, -102.8885) (-49.939, -103.5427) knots 0 0 0 0 1 1 1 1
  spline S198 degree 3 poles (-49.939, -103.5427) (-50.2978, -103.7327) (-50.4244, -103.7538) (-50.34, -103.6271) knots 0 0 0 0 1 1 1 1
  spline S199 degree 3 poles (-50.34, -103.6271) (-50.3189, -103.5849) (-50.3295, -103.4794) (-50.3822, -103.395) knots 0 0 0 0 1 1 1 1
  spline S200 degree 3 poles (-50.3822, -103.395) (-50.4561, -103.2789) (-50.6038, -103.3844) (-51.047, -103.8593) knots 0 0 0 0 1 1 1 1
  line L38 (-51.047, -103.8593) -> (-51.6168, -104.4819)
  line L39 (-51.6168, -104.4819) -> (-52.2183, -104.2497)
  spline S201 degree 3 poles (-52.2183, -104.2497) (-53.3051, -103.8487) (-54.8879, -103.5849) (-56.1858, -103.5955) knots 0 0 0 0 1 1 1 1
  spline S202 degree 3 poles (-56.1858, -103.5955) (-56.4496, -103.5955) (-56.7662, -103.5322) (-56.8823, -103.4478) knots 0 0 0 0 1 1 1 1
  spline S203 degree 3 poles (-56.8823, -103.4478) (-57.1988, -103.2473) (-57.5576, -102.4559) (-57.5576, -101.9916) knots 0 0 0 0 1 1 1 1
  spline S204 degree 3 poles (-57.5576, -101.9916) (-57.5576, -101.5378) (-57.6948, -101.4956) (-57.9269, -101.8544) knots 0 0 0 0 1 1 1 1
  spline S205 degree 3 poles (-57.3888, -103.1417) (-57.2832, -103.3106) (-57.1355, -103.49) (-57.0616, -103.5322) knots 0 0 0 0 1 1 1 1
  spline S206 degree 3 poles (-57.0616, -103.5322) (-56.8401, -103.6693) (-56.9034, -103.8171) (-57.1988, -103.8171) knots 0 0 0 0 1 1 1 1
  spline S207 degree 3 poles (-57.1988, -103.8171) (-57.5787, -103.8171) (-58.0852, -103.2895) (-58.0852, -102.8885) knots 0 0 0 0 1 1 1 1
  spline S208 degree 3 poles (-58.0852, -102.8885) (-58.0852, -102.7197) (-58.0008, -102.3926) (-57.9058, -102.171) knots 0 0 0 0 1 1 1 1
  line L40 (-57.9058, -102.171) -> (-57.7264, -101.7594)
  line L41 (-57.7264, -101.7594) -> (-57.6526, -102.2976)
  spline S209 degree 3 poles (-57.6526, -102.2976) (-57.6209, -102.593) (-57.4943, -102.9729) (-57.3888, -103.1417) knots 0 0 0 0 1 1 1 1
  spline S210 degree 3 poles (-45.9293, -103.5322) (-45.2856, -103.8171) (-44.9057, -104.5979) (-44.8952, -105.632) knots 0 0 0 0 1 1 1 1
  line L42 (-44.8952, -105.632) -> (-44.8952, -106.0225)
  line L43 (-44.8952, -106.0225) -> (-45.4755, -105.9591)
  spline S211 degree 3 poles (-45.4755, -105.9591) (-46.2247, -105.8853) (-46.3935, -106.0013) (-46.2458, -106.5289) knots 0 0 0 0 1 1 1 1
  spline S212 degree 3 poles (-46.2458, -106.5289) (-46.1192, -106.9932) (-46.2036, -107.352) (-46.5307, -107.7424) knots 0 0 0 0 1 1 1 1
  spline S213 degree 3 poles (-46.5307, -107.7424) (-46.8051, -108.0695) (-46.784, -108.3017) (-46.4674, -108.4705) knots 0 0 0 0 1 1 1 1
  spline S214 degree 3 poles (-46.4674, -108.4705) (-46.2775, -108.5655) (-46.2669, -108.5444) (-46.3302, -108.2806) knots 0 0 0 0 1 1 1 1
  spline S215 degree 3 poles (-46.3302, -108.2806) (-46.3619, -108.1223) (-46.4041, -107.9218) (-46.4358, -107.848) knots 0 0 0 0 1 1 1 1
  spline S216 degree 3 poles (-46.4358, -107.848) (-46.4569, -107.7846) (-46.4147, -107.7213) (-46.3408, -107.7213) knots 0 0 0 0 1 1 1 1
  spline S217 degree 3 poles (-46.3408, -107.7213) (-46.2353, -107.7213) (-46.1931, -108.154) (-46.2564, -108.6288) knots 0 0 0 0 1 1 1 1
  spline S218 degree 3 poles (-46.2564, -108.6288) (-46.2669, -108.7238) (-46.6996, -108.9876) (-46.8473, -108.9876) knots 0 0 0 0 1 1 1 1
  spline S219 degree 3 poles (-46.8473, -108.9876) (-46.8684, -108.9876) (-46.9845, -108.8293) (-47.1005, -108.6288) knots 0 0 0 0 1 1 1 1
  spline S220 degree 3 poles (-47.1005, -108.6288) (-47.2272, -108.4389) (-47.5859, -107.9535) (-47.9025, -107.5525) knots 0 0 0 0 1 1 1 1
  spline S221 degree 3 poles (-47.9025, -107.5525) (-48.2718, -107.0882) (-48.4406, -106.7927) (-48.3773, -106.7294) knots 0 0 0 0 1 1 1 1
  spline S222 degree 3 poles (-48.3773, -106.7294) (-48.2085, -106.5606) (-48.2613, -106.2651) (-48.4934, -106.0541) knots 0 0 0 0 1 1 1 1
  line L44 (-48.4934, -106.0541) -> (-48.7044, -105.8431)
  line L45 (-48.7044, -105.8431) -> (-48.4406, -105.7798)
  spline S223 degree 3 poles (-48.4406, -105.7798) (-48.2929, -105.7481) (-48.1663, -105.6531) (-48.1663, -105.5687) knots 0 0 0 0 1 1 1 1
  spline S224 degree 3 poles (-48.1663, -105.5687) (-48.1663, -105.3577) (-48.5778, -104.8723) (-48.7783, -104.8617) knots 0 0 0 0 1 1 1 1
  spline S225 degree 3 poles (-48.7783, -104.8617) (-49.116, -104.8406) (-48.3246, -104.6823) (-47.797, -104.6718) knots 0 0 0 0 1 1 1 1
  spline S226 degree 3 poles (-47.797, -104.6718) (-47.1638, -104.6612) (-46.5518, -104.8195) (-46.3724, -105.0306) knots 0 0 0 0 1 1 1 1
  spline S227 degree 3 poles (-46.3724, -105.0306) (-46.2986, -105.115) (-46.2036, -105.3471) (-46.1508, -105.5371) knots 0 0 0 0 1 1 1 1
  spline S228 degree 3 poles (-46.1508, -105.5371) (-46.0664, -105.8536) (-46.0664, -105.8536) (-46.1086, -105.4526) knots 0 0 0 0 1 1 1 1
  spline S229 degree 3 poles (-46.1086, -105.4526) (-46.1614, -104.9567) (-46.5413, -104.5979) (-47.09, -104.4924) knots 0 0 0 0 1 1 1 1
  spline S230 degree 3 poles (-47.09, -104.4924) (-47.607, -104.3974) (-48.5778, -104.503) (-49.0632, -104.7246) knots 0 0 0 0 1 1 1 1
  line L46 (-49.0632, -104.7246) -> (-49.4853, -104.9145)
  line L47 (-49.4853, -104.9145) -> (-49.0738, -104.9884)
  spline S231 degree 3 poles (-49.0738, -104.9884) (-48.8311, -105.0306) (-48.5673, -105.1572) (-48.4617, -105.2944) knots 0 0 0 0 1 1 1 1
  spline S232 degree 3 poles (-48.4617, -105.2944) (-48.2613, -105.5371) (-48.2613, -105.5371) (-48.6411, -105.7059) knots 0 0 0 0 1 1 1 1
  line L48 (-48.6411, -105.7059) -> (-49.021, -105.8747)
  line L49 (-49.021, -105.8747) -> (-48.7044, -106.0647)
  spline S233 degree 3 poles (-48.7044, -106.0647) (-48.3457, -106.2757) (-48.2824, -106.5289) (-48.5462, -106.6345) knots 0 0 0 0 1 1 1 1
  spline S234 degree 3 poles (-48.5462, -106.6345) (-48.6517, -106.6767) (-48.8944, -106.5184) (-49.2531, -106.1596) knots 0 0 0 0 1 1 1 1
  spline S235 degree 3 poles (-49.2531, -106.1596) (-49.5592, -105.8747) (-50.1712, -105.3893) (-50.6249, -105.1044) knots 0 0 0 0 1 1 1 1
  line L50 (-50.6249, -105.1044) -> (-51.448, -104.5663)
  line L51 (-51.448, -104.5663) -> (-50.9626, -104.0281)
  spline S236 degree 3 poles (-50.9626, -104.0281) (-50.5194, -103.5322) (-50.4877, -103.5111) (-50.4877, -103.7643) knots 0 0 0 0 1 1 1 1
  line L52 (-50.4877, -103.7643) -> (-50.4877, -104.0281)
  line L53 (-50.4877, -104.0281) -> (-50.0445, -103.8065)
  spline S237 degree 3 poles (-50.0445, -103.8065) (-49.116, -103.3317) (-48.9049, -103.2895) (-47.5859, -103.3317) knots 0 0 0 0 1 1 1 1
  spline S238 degree 3 poles (-47.5859, -103.3317) (-46.7207, -103.3528) (-46.1931, -103.4161) (-45.9293, -103.5322) knots 0 0 0 0 1 1 1 1
  spline S239 degree 3 poles (-62.211, -103.8804) (-61.8312, -104.0387) (-61.4724, -104.1969) (-61.4091, -104.2497) knots 0 0 0 0 1 1 1 1
  spline S240 degree 3 poles (-61.4091, -104.2497) (-61.2191, -104.4291) (-61.1242, -104.3447) (-61.1875, -104.0492) knots 0 0 0 0 1 1 1 1
  line L54 (-61.1875, -104.0492) -> (-61.2508, -103.7643)
  line L55 (-61.2508, -103.7643) -> (-61.0187, -104.0387)
  spline S241 degree 3 poles (-61.0187, -104.0387) (-60.8815, -104.1969) (-60.6388, -104.4396) (-60.4594, -104.5874) knots 0 0 0 0 1 1 1 1
  line L56 (-60.4594, -104.5874) -> (-60.1428, -104.8512)
  line L57 (-60.1428, -104.8512) -> (-61.082, -105.2838)
  spline S242 degree 3 poles (-61.082, -105.2838) (-61.905, -105.6637) (-62.8442, -106.2968) (-63.0658, -106.6028) knots 0 0 0 0 1 1 1 1
  spline S243 degree 3 poles (-63.0658, -106.6028) (-63.108, -106.6661) (-63.224, -106.6345) (-63.3612, -106.5078) knots 0 0 0 0 1 1 1 1
  line L58 (-63.3612, -106.5078) -> (-63.5934, -106.2968)
  line L59 (-63.5934, -106.2968) -> (-63.3612, -106.1174)
  spline S244 degree 3 poles (-63.3612, -106.1174) (-63.2346, -106.0119) (-63.0658, -105.9275) (-62.9813, -105.9275) knots 0 0 0 0 1 1 1 1
  spline S245 degree 3 poles (-62.9813, -105.9275) (-62.6753, -105.9275) (-62.8442, -105.727) (-63.2029, -105.6531) knots 0 0 0 0 1 1 1 1
  spline S246 degree 3 poles (-63.2029, -105.6531) (-63.414, -105.6215) (-63.5617, -105.5371) (-63.5406, -105.4737) knots 0 0 0 0 1 1 1 1
  spline S247 degree 3 poles (-63.5406, -105.4737) (-63.4773, -105.2838) (-63.0024, -104.9672) (-62.7492, -104.9461) knots 0 0 0 0 1 1 1 1
  spline S248 degree 3 poles (-62.7492, -104.9461) (-62.4221, -104.925) (-62.4537, -104.7879) (-62.802, -104.6929) knots 0 0 0 0 1 1 1 1
  spline S249 degree 3 poles (-62.802, -104.6929) (-63.4456, -104.5346) (-64.8174, -104.6401) (-65.2922, -104.8828) knots 0 0 0 0 1 1 1 1
  spline S250 degree 3 poles (-65.2922, -104.8828) (-65.7671, -105.1255) (-65.8937, -105.3155) (-65.8937, -105.7587) knots 0 0 0 0 1 1 1 1
  spline S251 degree 3 poles (-65.8937, -105.7587) (-65.8937, -106.0541) (-65.862, -106.1385) (-65.7987, -106.0436) knots 0 0 0 0 1 1 1 1
  spline S252 degree 3 poles (-65.7987, -106.0436) (-65.746, -105.9591) (-65.7143, -105.7903) (-65.7354, -105.6531) knots 0 0 0 0 1 1 1 1
  spline S253 degree 3 poles (-65.7354, -105.6531) (-65.746, -105.516) (-65.6827, -105.3366) (-65.5877, -105.2627) knots 0 0 0 0 1 1 1 1
  spline S254 degree 3 poles (-65.5877, -105.2627) (-65.2817, -104.9884) (-64.3848, -104.7668) (-63.6356, -104.7668) knots 0 0 0 0 1 1 1 1
  line L60 (-63.6356, -104.7668) -> (-62.8864, -104.7668)
  line L61 (-62.8864, -104.7668) -> (-63.2135, -104.9672)
  spline S255 degree 3 poles (-63.2135, -104.9672) (-63.72, -105.2838) (-63.931, -105.7164) (-63.5722, -105.7164) knots 0 0 0 0 1 1 1 1
  spline S256 degree 3 poles (-63.5722, -105.7164) (-63.4667, -105.7164) (-63.3401, -105.7587) (-63.3084, -105.822) knots 0 0 0 0 1 1 1 1
  spline S257 degree 3 poles (-63.3084, -105.822) (-63.2768, -105.8747) (-63.2873, -105.9275) (-63.3507, -105.9275) knots 0 0 0 0 1 1 1 1
  spline S258 degree 3 poles (-63.3507, -105.9275) (-63.414, -105.9275) (-63.5089, -106.0225) (-63.5722, -106.1491) knots 0 0 0 0 1 1 1 1
  spline S259 degree 3 poles (-63.5722, -106.1491) (-63.6672, -106.3179) (-63.6567, -106.4129) (-63.5089, -106.5712) knots 0 0 0 0 1 1 1 1
  spline S260 degree 3 poles (-63.5089, -106.5712) (-63.3401, -106.7611) (-63.3401, -106.7822) (-63.5195, -106.9827) knots 0 0 0 0 1 1 1 1
  spline S261 degree 3 poles (-63.5195, -106.9827) (-63.7516, -107.2359) (-63.8783, -107.1726) (-63.6672, -106.9088) knots 0 0 0 0 1 1 1 1
  spline S262 degree 3 poles (-63.6672, -106.9088) (-63.53, -106.74) (-63.5406, -106.7294) (-63.7094, -106.8666) knots 0 0 0 0 1 1 1 1
  spline S263 degree 3 poles (-63.7094, -106.8666) (-63.8149, -106.951) (-63.8783, -107.0777) (-63.8466, -107.1515) knots 0 0 0 0 1 1 1 1
  spline S264 degree 3 poles (-63.8466, -107.1515) (-63.8149, -107.2254) (-63.931, -107.4575) (-64.0999, -107.6686) knots 0 0 0 0 1 1 1 1
  spline S265 degree 3 poles (-64.0999, -107.6686) (-64.2581, -107.8691) (-64.5536, -108.2806) (-64.733, -108.5655) knots 0 0 0 0 1 1 1 1
  spline S266 degree 3 poles (-64.733, -108.5655) (-65.039, -109.0403) (-65.0812, -109.072) (-65.3239, -108.9665) knots 0 0 0 0 1 1 1 1
  spline S267 degree 3 poles (-65.3239, -108.9665) (-65.5982, -108.8398) (-65.6299, -108.766) (-65.4716, -108.6077) knots 0 0 0 0 1 1 1 1
  spline S268 degree 3 poles (-65.4716, -108.6077) (-65.4083, -108.5444) (-65.44, -108.2595) (-65.5771, -107.7846) knots 0 0 0 0 1 1 1 1
  spline S269 degree 3 poles (-65.5771, -107.7846) (-65.6932, -107.3837) (-65.7565, -107.0249) (-65.7354, -106.9721) knots 0 0 0 0 1 1 1 1
  spline S270 degree 3 poles (-65.7354, -106.9721) (-65.7038, -106.9299) (-65.7354, -106.8561) (-65.7987, -106.8139) knots 0 0 0 0 1 1 1 1
  spline S271 degree 3 poles (-65.7987, -106.8139) (-65.9465, -106.7189) (-65.862, -107.3942) (-65.6404, -108.0379) knots 0 0 0 0 1 1 1 1
  spline S272 degree 3 poles (-65.6404, -108.0379) (-65.5244, -108.3861) (-65.5244, -108.4705) (-65.651, -108.5971) knots 0 0 0 0 1 1 1 1
  spline S273 degree 3 poles (-65.651, -108.5971) (-65.8198, -108.7554) (-65.7776, -108.8187) (-65.3344, -109.1247) knots 0 0 0 0 1 1 1 1
  spline S274 degree 3 poles (-65.3344, -109.1247) (-65.1551, -109.2514) (-65.1551, -109.283) (-65.4189, -109.8634) knots 0 0 0 0 1 1 1 1
  spline S275 degree 3 poles (-65.4189, -109.8634) (-65.6721, -110.4121) (-65.7143, -110.4543) (-65.9254, -110.3488) knots 0 0 0 0 1 1 1 1
  spline S276 degree 3 poles (-65.9254, -110.3488) (-66.1258, -110.2327) (-66.1364, -110.2222) (-65.957, -110.085) knots 0 0 0 0 1 1 1 1
  spline S277 degree 3 poles (-65.957, -110.085) (-65.7776, -109.9584) (-65.7987, -109.9056) (-66.1997, -109.3463) knots 0 0 0 0 1 1 1 1
  spline S278 degree 3 poles (-66.1997, -109.3463) (-66.4424, -109.0192) (-66.6323, -108.671) (-66.6323, -108.5866) knots 0 0 0 0 1 1 1 1
  spline S279 degree 3 poles (-66.6323, -108.5866) (-66.6323, -108.5022) (-66.759, -108.2911) (-66.9067, -108.1118) knots 0 0 0 0 1 1 1 1
  spline S280 degree 3 poles (-66.9067, -108.1118) (-67.1599, -107.8163) (-67.1705, -107.7741) (-67.0017, -107.658) knots 0 0 0 0 1 1 1 1
  spline S281 degree 3 poles (-67.0017, -107.658) (-66.8434, -107.5419) (-66.8434, -107.4786) (-66.9489, -107.1304) knots 0 0 0 0 1 1 1 1
  spline S282 degree 3 poles (-66.9489, -107.1304) (-67.1177, -106.645) (-67.1177, -105.3893) (-66.9595, -104.809) knots 0 0 0 0 1 1 1 1
  spline S283 degree 3 poles (-66.9595, -104.809) (-66.8434, -104.3763) (-66.4318, -103.912) (-66.052, -103.7749) knots 0 0 0 0 1 1 1 1
  spline S284 degree 3 poles (-66.052, -103.7749) (-65.9359, -103.7327) (-65.5982, -103.6693) (-65.3133, -103.6377) knots 0 0 0 0 1 1 1 1
  spline S285 degree 3 poles (-65.3133, -103.6377) (-65.0179, -103.606) (-64.7646, -103.5533) (-64.733, -103.5322) knots 0 0 0 0 1 1 1 1
  spline S286 degree 3 poles (-64.733, -103.5322) (-64.5852, -103.3844) (-62.8547, -103.6271) (-62.211, -103.8804) knots 0 0 0 0 1 1 1 1
  line L62 (-45.5494, -106.3707) -> (-45.4228, -106.7189)
  line L63 (-45.4228, -106.7189) -> (-45.4755, -106.4023)
  line L64 (-45.4755, -106.4023) -> (-45.5283, -106.0858)
  line L65 (-45.5283, -106.0858) -> (-45.37, -106.3496)
  spline S287 degree 3 poles (-45.37, -106.3496) (-45.1484, -106.7294) (-45.1695, -106.8561) (-45.465, -106.8033) knots 0 0 0 0 1 1 1 1
  spline S288 degree 3 poles (-45.465, -106.8033) (-45.6549, -106.7611) (-45.7499, -106.6556) (-45.7921, -106.434) knots 0 0 0 0 1 1 1 1
  spline S289 degree 3 poles (-45.7921, -106.434) (-45.8448, -106.2124) (-45.8976, -106.1491) (-45.982, -106.2335) knots 0 0 0 0 1 1 1 1
  spline S290 degree 3 poles (-45.982, -106.2335) (-46.0559, -106.3074) (-46.0453, -106.3918) (-45.9504, -106.5078) knots 0 0 0 0 1 1 1 1
  spline S291 degree 3 poles (-45.9504, -106.5078) (-45.8765, -106.6028) (-45.8659, -106.6661) (-45.9293, -106.6661) knots 0 0 0 0 1 1 1 1
  spline S292 degree 3 poles (-45.9293, -106.6661) (-45.9926, -106.6661) (-46.0664, -106.5712) (-46.1086, -106.4551) knots 0 0 0 0 1 1 1 1
  spline S293 degree 3 poles (-46.1086, -106.4551) (-46.2775, -105.938) (-45.7288, -105.8642) (-45.5494, -106.3707) knots 0 0 0 0 1 1 1 1
  spline S294 degree 3 poles (-44.6736, -106.3285) (-44.5575, -106.4445) (-44.7685, -106.8772) (-44.9479, -106.8772) knots 0 0 0 0 1 1 1 1
  spline S295 degree 3 poles (-44.9479, -106.8772) (-45.0851, -106.8772) (-45.1379, -106.6978) (-45.0956, -106.3918) knots 0 0 0 0 1 1 1 1
  spline S296 degree 3 poles (-45.0956, -106.3918) (-45.0956, -106.3496) (-45.1484, -106.2757) (-45.2328, -106.2229) knots 0 0 0 0 1 1 1 1
  spline S297 degree 3 poles (-45.2328, -106.2229) (-45.3278, -106.1596) (-45.2645, -106.1491) (-45.0534, -106.1913) knots 0 0 0 0 1 1 1 1
  spline S298 degree 3 poles (-45.0534, -106.1913) (-44.8741, -106.2229) (-44.7052, -106.2863) (-44.6736, -106.3285) knots 0 0 0 0 1 1 1 1
  spline S299 degree 3 poles (-67.1599, -106.74) (-67.1599, -106.8455) (-67.1283, -107.0249) (-67.0966, -107.141) knots 0 0 0 0 1 1 1 1
  spline S300 degree 3 poles (-67.0966, -107.141) (-67.0544, -107.3204) (-67.1388, -107.4048) (-67.6031, -107.6158) knots 0 0 0 0 1 1 1 1